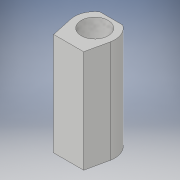
# Autodesk Inventor part: JlinearActuator1
Saved by Autodesk Inventor 2018 (Build 220112000, 112)
## iProperties
Created: 2020-04-10
Part Number: JlinearActuator1
Material: Generic
Document SubType Name: Modeling
Designer: Jesse R-B
Density: 1 g/cm^3
Appearance: Default
Author: Jesse R-B
Autodesk Inventor part; units mm, degrees
ref_plane "YZ Plane" through (0, 0, 0) normal (1, 0, 0) x (0, 1, 0)
ref_plane "XZ Plane" through (0, 0, 0) normal (0, 1, 0) x (-1, 0, 0)
ref_plane "XY Plane" through (0, 0, 0) normal (0, 0, 1) x (1, 0, 0)
sketch "Sketch1" plane through (0, 0, 0) normal (0, 1, 0) x (-1, 0, 0)
  line L0 (19.6595, 54.9113) -> (15.5413, 59.0295)
  arc A0 (15.5413, 59.0295) -> (13.0268, 60.071) centre (13.0268, 56.515) ccw
  line L1 (13.0268, 60.071) -> (-13.0268, 60.071)
  arc A1 (-13.0268, 60.071) -> (-15.5413, 59.0295) centre (-13.0268, 56.515) ccw
  line L2 (-15.5413, 59.0295) -> (-19.6595, 54.9113)
  arc A2 (-19.6595, 54.9113) -> (-20.701, 52.3968) centre (-17.145, 52.3968) ccw
  line L3 (-20.701, 52.3968) -> (-20.701, 0)
  arc A3 (-20.701, 0) -> (20.701, 0) centre (0, 0) ccw
  line L4 (20.701, 0) -> (20.701, 52.3968)
  arc A4 (20.701, 52.3968) -> (19.6595, 54.9113) centre (17.145, 52.3968) ccw
  arc A5 (8.4594, 23.8249) -> (8.3222, 23.1257) centre (8.7461, 23.4056) ccw
  arc A6 (8.4594, 23.8249) -> (14.6472, 39.3636) centre (0, 36.195) ccw
  line L5 (14.6472, 39.3636) -> (11.148, 55.5389)
  arc A7 (11.5371, 56.1429) -> (11.148, 55.5389) centre (11.6445, 55.6463) ccw
  line L6 (11.5371, 56.1429) -> (13.5232, 56.5725)
  arc A8 (14.1271, 56.1834) -> (13.5232, 56.5725) centre (13.6306, 56.076) ccw
  line L7 (14.1271, 56.1834) -> (17.6263, 40.0081)
  arc A9 (10.1516, 21.2896) -> (17.6263, 40.0081) centre (0, 36.195) ccw
  arc A10 (9.4417, 21.4297) -> (10.1516, 21.2896) centre (9.8656, 21.7095) ccw
  line L8 (9.4417, 21.4297) -> (8.3222, 23.1257)
  arc A11 (-13.5232, 56.5725) -> (-14.1271, 56.1834) centre (-13.6306, 56.076) ccw
  line L9 (-13.5232, 56.5725) -> (-11.5371, 56.1429)
  arc A12 (-11.148, 55.5389) -> (-11.5371, 56.1429) centre (-11.6445, 55.6463) ccw
  line L10 (-11.148, 55.5389) -> (-14.6472, 39.3636)
  arc A13 (-14.6472, 39.3636) -> (-8.4594, 23.8249) centre (0, 36.195) ccw
  arc A14 (-8.3222, 23.1257) -> (-8.4594, 23.8249) centre (-8.7461, 23.4056) ccw
  line L11 (-8.3222, 23.1257) -> (-9.4417, 21.4297)
  arc A15 (-10.1516, 21.2896) -> (-9.4417, 21.4297) centre (-9.8656, 21.7095) ccw
  arc A16 (-17.6263, 40.0081) -> (-10.1516, 21.2896) centre (0, 36.195) ccw
  line L12 (-17.6263, 40.0081) -> (-14.1271, 56.1834)
  circle A17 centre (0, 0) radius 20.193
  line L13 (11.148, 55.5389) -> (-11.148, 55.5389)
  line L14 (11.148, 55.5389) -> (14.6472, 39.3636)
  arc A18 (8.4594, 23.8249) -> (14.6472, 39.3636) centre (0, 36.195) ccw
  line L15 (-11.148, 55.5389) -> (-14.6472, 39.3636)
  arc A19 (-14.6472, 39.3636) -> (-8.4594, 23.8249) centre (0, 36.195) ccw
  line L16 (8.4594, 23.8249) -> (-8.4594, 23.8249)
  constraints: 38 point on circle, 34 end point, 20 centre point, 2 horizontal, 2 tangent, 1 concentric
extrude "Extrusion1" add sketch "Sketch1" along normal blind 76.2 contours L16 A13 L10 L13 L5 A6
sketch "Sketch2" plane through (0, 76.2, 0) normal (0, 1, 0) x (1, 0, 0)
  line L0 (-11.148, -55.5389) -> (11.148, -55.5389) projected
  line L1 (11.148, -55.5389) -> (14.6472, -39.3636) projected
  arc A0 (14.6472, -39.3636) -> (8.4594, -23.8249) centre (0, -36.195) ccw projected
  line L2 (8.4594, -23.8249) -> (-8.4594, -23.8249) projected
  arc A1 (-8.4594, -23.8249) -> (-14.6472, -39.3636) centre (0, -36.195) ccw projected
  line L3 (-14.6472, -39.3636) -> (-11.148, -55.5389) projected
  circle A2 centre (0, -36.195) radius 9.9695
  point P0 (0, 0)
  dimension "d2" = 19.939
  constraints: 1 centre point, 1 coincident
  measures "d2" diameter of A2
extrude "Extrusion2" cut sketch "Sketch2" against normal blind 76.2 contours A2
body "Solid1"
